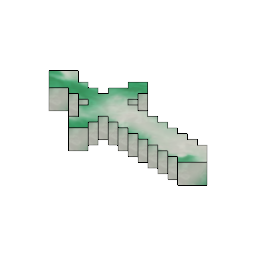
minecraftdiamondsword for big CNC schetch straight_v1 (Autodesk Fusion 360 design; units mm, degrees)
Autodesk Fusion 360 part; units mm, degrees
sketch "big huge diamond sword" plane through (0, 0, 0) normal (0, 0, 1) x (1, 0, 0)
  line L0 (-48.4562, -24.0547) -> (-40.4562, -24.0547)
  line L1 (-40.4562, -24.0547) -> (-40.4562, -16.0547)
  line L2 (-40.4562, -16.0547) -> (-48.4562, -16.0547)
  line L3 (-48.4562, -16.0547) -> (-48.4562, -24.0547)
  line L4 (-40.4562, -24.0547) -> (-32.4562, -24.0547)
  line L5 (-32.4562, -24.0547) -> (-32.4562, -16.0547)
  line L6 (-32.4562, -16.0547) -> (-40.4562, -16.0547)
  line L7 (-40.4562, -16.0547) -> (-40.4562, -24.0547)
  line L8 (-32.4562, -24.0547) -> (-24.4562, -24.0547)
  line L9 (-24.4562, -24.0547) -> (-24.4562, -16.0547)
  line L10 (-32.4562, -16.0547) -> (-32.4562, -24.0547)
  line L11 (-48.4562, -16.0547) -> (-40.4562, -16.0547)
  line L12 (-40.4562, -16.0547) -> (-40.4562, -8.0547)
  line L13 (-40.4562, -8.0547) -> (-48.4562, -8.0547)
  line L14 (-48.4562, -8.0547) -> (-48.4562, -16.0547)
  line L15 (-40.4562, -8.0547) -> (-32.4562, -8.0547)
  line L16 (-32.4562, -8.0547) -> (-32.4562, -16.0547)
  line L17 (-32.4562, -16.0547) -> (-40.4562, -16.0547)
  line L18 (-40.4562, -16.0547) -> (-40.4562, -8.0547)
  line L19 (-48.4562, -8.0547) -> (-40.4562, -8.0547)
  line L20 (-40.4562, -8.0547) -> (-40.4562, -0.0547)
  line L21 (-40.4562, -0.0547) -> (-48.4562, -0.0547)
  line L22 (-48.4562, -0.0547) -> (-48.4562, -8.0547)
  line L23 (-40.4562, -8.0547) -> (-32.4562, -8.0547)
  line L24 (-32.4562, -8.0547) -> (-32.4562, -0.0547)
  line L25 (-32.4562, -0.0547) -> (-40.4562, -0.0547)
  line L26 (-40.4562, -0.0547) -> (-40.4562, -8.0547)
  line L27 (-32.4562, -8.0547) -> (-24.4562, -8.0547)
  line L28 (-24.4562, -8.0547) -> (-24.4562, -16.0547)
  line L29 (-24.4562, -16.0547) -> (-32.4562, -16.0547)
  line L30 (-32.4562, -16.0547) -> (-32.4562, -8.0547)
  line L31 (-32.4562, -8.0547) -> (-24.4562, -8.0547)
  line L32 (-24.4562, -8.0547) -> (-24.4562, -0.0547)
  line L33 (-24.4562, -0.0547) -> (-32.4562, -0.0547)
  line L34 (-32.4562, -0.0547) -> (-32.4562, -8.0547)
  line L35 (-32.4562, -0.0547) -> (-24.4562, -0.0547)
  line L36 (-24.4562, -0.0547) -> (-24.4562, 7.9453)
  line L37 (-24.4562, 7.9453) -> (-32.4562, 7.9453)
  line L38 (-32.4562, 7.9453) -> (-32.4562, -0.0547)
  line L39 (-24.4562, -0.0547) -> (-16.4562, -0.0547)
  line L40 (-16.4562, -0.0547) -> (-16.4562, -8.0547)
  line L41 (-16.4562, -8.0547) -> (-24.4562, -8.0547)
  line L42 (-24.4562, -8.0547) -> (-24.4562, -0.0547)
  line L43 (-24.4562, -0.0547) -> (-16.4562, -0.0547)
  line L44 (-16.4562, -0.0547) -> (-16.4562, 7.9453)
  line L45 (-16.4562, 7.9453) -> (-24.4562, 7.9453)
  line L46 (-24.4562, 7.9453) -> (-24.4562, -0.0547)
  line L47 (-24.4562, 7.9453) -> (-16.4562, 7.9453)
  line L48 (-16.4562, 7.9453) -> (-16.4562, 15.9453)
  line L49 (-16.4562, 15.9453) -> (-24.4562, 15.9453)
  line L50 (-24.4562, 15.9453) -> (-24.4562, 7.9453)
  line L51 (-16.4562, 7.9453) -> (-8.4562, 7.9453)
  line L52 (-8.4562, -0.0547) -> (-16.4562, -0.0547)
  line L53 (-16.4562, -0.0547) -> (-16.4562, 7.9453)
  line L54 (-16.4562, 7.9453) -> (-8.4562, 7.9453)
  line L55 (-8.4562, 7.9453) -> (-8.4562, 15.9453)
  line L56 (-8.4562, 15.9453) -> (-16.4562, 15.9453)
  line L57 (-16.4562, 15.9453) -> (-16.4562, 7.9453)
  line L58 (-16.4562, 15.9453) -> (-8.4562, 15.9453)
  line L59 (-8.4562, 15.9453) -> (-8.4562, 23.9453)
  line L60 (-8.4562, 23.9453) -> (-16.4562, 23.9453)
  line L61 (-16.4562, 23.9453) -> (-16.4562, 15.9453)
  line L62 (-16.4562, 23.9453) -> (-24.4562, 23.9453)
  line L63 (-24.4562, 23.9453) -> (-24.4562, 31.9453)
  line L64 (-24.4562, 31.9453) -> (-16.4562, 31.9453)
  line L65 (-16.4562, 31.9453) -> (-16.4562, 23.9453)
  line L66 (-24.4562, 31.9453) -> (-16.4562, 31.9453)
  line L67 (-16.4562, 31.9453) -> (-16.4562, 39.9453)
  line L68 (-16.4562, 39.9453) -> (-24.4562, 39.9453)
  line L69 (-24.4562, 39.9453) -> (-24.4562, 31.9453)
  line L70 (-24.4562, 39.9453) -> (-32.4562, 39.9453)
  line L71 (-32.4562, 39.9453) -> (-32.4562, 47.9453)
  line L72 (-32.4562, 47.9453) -> (-24.4562, 47.9453)
  line L73 (-24.4562, 47.9453) -> (-24.4562, 39.9453)
  line L74 (-32.4562, 47.9453) -> (-24.4562, 47.9453)
  line L75 (-24.4562, 47.9453) -> (-24.4562, 55.9453)
  line L76 (-24.4562, 55.9453) -> (-32.4562, 55.9453)
  line L77 (-32.4562, 55.9453) -> (-32.4562, 47.9453)
  line L78 (-24.4562, 47.9453) -> (-16.4562, 47.9453)
  line L79 (-16.4562, 47.9453) -> (-16.4562, 55.9453)
  line L80 (-16.4562, 55.9453) -> (-24.4562, 55.9453)
  line L81 (-24.4562, 55.9453) -> (-24.4562, 47.9453)
  line L82 (-24.4562, 39.9453) -> (-16.4562, 39.9453)
  line L83 (-16.4562, 39.9453) -> (-16.4562, 47.9453)
  line L84 (-16.4562, 47.9453) -> (-24.4562, 47.9453)
  line L85 (-24.4562, 47.9453) -> (-24.4562, 39.9453)
  line L86 (-16.4562, 47.9453) -> (-8.4562, 47.9453)
  line L87 (-8.4562, 47.9453) -> (-8.4562, 39.9453)
  line L88 (-8.4562, 39.9453) -> (-16.4562, 39.9453)
  line L89 (-16.4562, 39.9453) -> (-16.4562, 47.9453)
  line L90 (-16.4562, 39.9453) -> (-8.4562, 39.9453)
  line L91 (-8.4562, 39.9453) -> (-8.4562, 31.9453)
  line L92 (-8.4562, 31.9453) -> (-16.4562, 31.9453)
  line L93 (-16.4562, 31.9453) -> (-16.4562, 39.9453)
  line L94 (-16.4562, 23.9453) -> (-8.4562, 23.9453)
  line L95 (-8.4562, 23.9453) -> (-8.4562, 31.9453)
  line L96 (-8.4562, 31.9453) -> (-16.4562, 31.9453)
  line L97 (-16.4562, 31.9453) -> (-16.4562, 23.9453)
  line L98 (-8.4562, 7.9453) -> (-0.4562, 7.9453)
  line L99 (-8.4562, -0.0547) -> (-8.4562, 7.9453)
  line L100 (-8.4562, 15.9453) -> (-0.4562, 15.9453)
  line L101 (-0.4562, 15.9453) -> (-0.4562, 7.9453)
  line L102 (-8.4562, 7.9453) -> (-8.4562, 15.9453)
  line L103 (-8.4562, 23.9453) -> (-0.4562, 23.9453)
  line L104 (-0.4562, 23.9453) -> (-0.4562, 15.9453)
  line L105 (-0.4562, 15.9453) -> (-8.4562, 15.9453)
  line L106 (-8.4562, 15.9453) -> (-8.4562, 23.9453)
  line L107 (-0.4562, 7.9453) -> (7.5438, 7.9453)
  line L108 (7.5438, 7.9453) -> (7.5438, -0.0547)
  line L109 (7.5438, -0.0547) -> (-0.4562, -0.0547)
  line L110 (-0.4562, -0.0547) -> (-0.4562, 7.9453)
  line L111 (-0.4562, 7.9453) -> (7.5438, 7.9453)
  line L112 (7.5438, 7.9453) -> (7.5438, 15.9453)
  line L113 (7.5438, 15.9453) -> (-0.4562, 15.9453)
  line L114 (-0.4562, 15.9453) -> (-0.4562, 7.9453)
  line L115 (7.5438, 7.9453) -> (15.5438, 7.9453)
  line L116 (15.5438, 7.9453) -> (15.5438, -0.0547)
  line L117 (15.5438, -0.0547) -> (7.5438, -0.0547)
  line L118 (7.5438, -0.0547) -> (7.5438, 7.9453)
  line L119 (15.5438, -0.0547) -> (23.5438, -0.0547)
  line L120 (23.5438, -0.0547) -> (23.5438, 7.9453)
  line L121 (23.5438, 7.9453) -> (15.5438, 7.9453)
  line L122 (15.5438, 7.9453) -> (15.5438, -0.0547)
  line L123 (23.5438, -0.0547) -> (31.5438, -0.0547)
  line L124 (31.5438, -0.0547) -> (31.5438, 7.9453)
  line L125 (31.5438, 7.9453) -> (23.5438, 7.9453)
  line L126 (23.5438, 7.9453) -> (23.5438, -0.0547)
  line L127 (15.5438, -0.0547) -> (23.5438, -0.0547)
  line L128 (23.5438, -0.0547) -> (23.5438, -8.0547)
  line L129 (23.5438, -8.0547) -> (15.5438, -8.0547)
  line L130 (15.5438, -8.0547) -> (15.5438, -0.0547)
  line L131 (23.5438, -0.0547) -> (31.5438, -0.0547)
  line L132 (31.5438, -0.0547) -> (31.5438, -8.0547)
  line L133 (31.5438, -8.0547) -> (23.5438, -8.0547)
  line L134 (23.5438, -8.0547) -> (23.5438, -0.0547)
  line L135 (-8.4562, 31.9453) -> (-0.4562, 31.9453)
  line L136 (-0.4562, 31.9453) -> (-0.4562, 23.9453)
  line L137 (-0.4562, 23.9453) -> (-8.4562, 23.9453)
  line L138 (-8.4562, 23.9453) -> (-8.4562, 31.9453)
  line L139 (-0.4562, 23.9453) -> (7.5438, 23.9453)
  line L140 (7.5438, 23.9453) -> (7.5438, 15.9453)
  line L141 (7.5438, 15.9453) -> (-0.4562, 15.9453)
  line L142 (-0.4562, 15.9453) -> (-0.4562, 23.9453)
  line L143 (-8.4562, 39.9453) -> (-0.4562, 39.9453)
  line L144 (-0.4562, 39.9453) -> (-0.4562, 31.9453)
  line L145 (-0.4562, 31.9453) -> (-8.4562, 31.9453)
  line L146 (-8.4562, 31.9453) -> (-8.4562, 39.9453)
  line L147 (-0.4562, 31.9453) -> (7.5438, 31.9453)
  line L148 (7.5438, 31.9453) -> (7.5438, 23.9453)
  line L149 (7.5438, 23.9453) -> (-0.4562, 23.9453)
  line L150 (-0.4562, 23.9453) -> (-0.4562, 31.9453)
  line L151 (-0.4562, 39.9453) -> (7.5438, 39.9453)
  line L152 (7.5438, 39.9453) -> (7.5438, 31.9453)
  line L153 (7.5438, 31.9453) -> (-0.4562, 31.9453)
  line L154 (-0.4562, 31.9453) -> (-0.4562, 39.9453)
  line L155 (7.5438, 15.9453) -> (15.5438, 15.9453)
  line L156 (15.5438, 15.9453) -> (15.5438, 7.9453)
  line L157 (15.5438, 7.9453) -> (7.5438, 7.9453)
  line L158 (7.5438, 7.9453) -> (7.5438, 15.9453)
  line L159 (15.5438, 15.9453) -> (23.5438, 15.9453)
  line L160 (23.5438, 15.9453) -> (23.5438, 7.9453)
  line L161 (23.5438, 7.9453) -> (15.5438, 7.9453)
  line L162 (15.5438, 7.9453) -> (15.5438, 15.9453)
  line L163 (7.5438, 23.9453) -> (15.5438, 23.9453)
  line L164 (15.5438, 23.9453) -> (15.5438, 15.9453)
  line L165 (15.5438, 15.9453) -> (7.5438, 15.9453)
  line L166 (7.5438, 15.9453) -> (7.5438, 23.9453)
  line L167 (7.5438, 31.9453) -> (15.5438, 31.9453)
  line L168 (15.5438, 31.9453) -> (15.5438, 23.9453)
  line L169 (15.5438, 23.9453) -> (7.5438, 23.9453)
  line L170 (7.5438, 23.9453) -> (7.5438, 31.9453)
  line L171 (15.5438, 23.9453) -> (7.5438, 23.9453)
  line L172 (7.5438, 23.9453) -> (7.5438, 31.9453)
  line L173 (7.5438, 31.9453) -> (15.5438, 31.9453)
  line L174 (15.5438, 31.9453) -> (15.5438, 23.9453)
  line L175 (15.5438, 23.9453) -> (23.5438, 23.9453)
  line L176 (23.5438, 23.9453) -> (23.5438, 31.9453)
  line L177 (23.5438, 31.9453) -> (15.5438, 31.9453)
  line L178 (15.5438, 31.9453) -> (15.5438, 23.9453)
  line L179 (7.5438, 31.9453) -> (15.5438, 31.9453)
  line L180 (15.5438, 31.9453) -> (15.5438, 39.9453)
  line L181 (15.5438, 39.9453) -> (7.5438, 39.9453)
  line L182 (7.5438, 39.9453) -> (7.5438, 31.9453)
  line L183 (15.5438, 31.9453) -> (23.5438, 31.9453)
  line L184 (23.5438, 31.9453) -> (23.5438, 39.9453)
  line L185 (23.5438, 39.9453) -> (15.5438, 39.9453)
  line L186 (15.5438, 39.9453) -> (15.5438, 31.9453)
  line L187 (23.5438, 31.9453) -> (31.5438, 31.9453)
  line L188 (31.5438, 31.9453) -> (31.5438, 39.9453)
  line L189 (31.5438, 39.9453) -> (23.5438, 39.9453)
  line L190 (23.5438, 39.9453) -> (23.5438, 31.9453)
  line L191 (-0.4562, 39.9453) -> (7.5438, 39.9453)
  line L192 (7.5438, 39.9453) -> (7.5438, 47.9453)
  line L193 (7.5438, 47.9453) -> (-0.4562, 47.9453)
  line L194 (-0.4562, 47.9453) -> (-0.4562, 39.9453)
  line L195 (7.5438, 39.9453) -> (15.5438, 39.9453)
  line L196 (15.5438, 39.9453) -> (15.5438, 47.9453)
  line L197 (15.5438, 47.9453) -> (7.5438, 47.9453)
  line L198 (7.5438, 47.9453) -> (7.5438, 39.9453)
  line L199 (15.5438, 47.9453) -> (7.5438, 47.9453)
  line L200 (7.5438, 47.9453) -> (7.5438, 55.9453)
  line L201 (7.5438, 55.9453) -> (15.5438, 55.9453)
  line L202 (15.5438, 55.9453) -> (15.5438, 47.9453)
  line L203 (15.5438, 39.9453) -> (23.5438, 39.9453)
  line L204 (23.5438, 39.9453) -> (23.5438, 47.9453)
  line L205 (23.5438, 47.9453) -> (15.5438, 47.9453)
  line L206 (15.5438, 47.9453) -> (15.5438, 39.9453)
  line L207 (15.5438, 47.9453) -> (23.5438, 47.9453)
  line L208 (23.5438, 47.9453) -> (23.5438, 55.9453)
  line L209 (23.5438, 55.9453) -> (15.5438, 55.9453)
  line L210 (15.5438, 55.9453) -> (15.5438, 47.9453)
  line L211 (23.5438, 39.9453) -> (31.5438, 39.9453)
  line L212 (31.5438, 39.9453) -> (31.5438, 47.9453)
  line L213 (31.5438, 47.9453) -> (23.5438, 47.9453)
  line L214 (23.5438, 47.9453) -> (23.5438, 39.9453)
  line L215 (15.5438, 55.9453) -> (23.5438, 55.9453)
  line L216 (23.5438, 55.9453) -> (23.5438, 63.9453)
  line L217 (23.5438, 63.9453) -> (15.5438, 63.9453)
  line L218 (15.5438, 63.9453) -> (15.5438, 55.9453)
  line L219 (31.5438, 39.9453) -> (39.5438, 39.9453)
  line L220 (39.5438, 39.9453) -> (39.5438, 47.9453)
  line L221 (39.5438, 47.9453) -> (31.5438, 47.9453)
  line L222 (31.5438, 47.9453) -> (31.5438, 39.9453)
  line L223 (23.5438, 47.9453) -> (31.5438, 47.9453)
  line L224 (31.5438, 47.9453) -> (31.5438, 55.9453)
  line L225 (31.5438, 55.9453) -> (23.5438, 55.9453)
  line L226 (23.5438, 55.9453) -> (23.5438, 47.9453)
  line L227 (31.5438, 55.9453) -> (39.5438, 55.9453)
  line L228 (39.5438, 55.9453) -> (39.5438, 63.9453)
  line L229 (39.5438, 63.9453) -> (31.5438, 63.9453)
  line L230 (31.5438, 63.9453) -> (31.5438, 55.9453)
  line L231 (31.5438, 55.9453) -> (23.5438, 55.9453)
  line L232 (23.5438, 55.9453) -> (23.5438, 63.9453)
  line L233 (23.5438, 63.9453) -> (31.5438, 63.9453)
  line L234 (31.5438, 63.9453) -> (31.5438, 55.9453)
  line L235 (31.5438, 55.9453) -> (39.5438, 55.9453)
  line L236 (39.5438, 55.9453) -> (39.5438, 47.9453)
  line L237 (39.5438, 47.9453) -> (31.5438, 47.9453)
  line L238 (31.5438, 47.9453) -> (31.5438, 55.9453)
  line L239 (23.5438, 63.9453) -> (31.5438, 63.9453)
  line L240 (31.5438, 63.9453) -> (31.5438, 71.9453)
  line L241 (31.5438, 71.9453) -> (23.5438, 71.9453)
  line L242 (23.5438, 71.9453) -> (23.5438, 63.9453)
  line L243 (31.5438, 63.9453) -> (39.5438, 63.9453)
  line L244 (39.5438, 63.9453) -> (39.5438, 71.9453)
  line L245 (39.5438, 71.9453) -> (31.5438, 71.9453)
  line L246 (31.5438, 71.9453) -> (31.5438, 63.9453)
  line L247 (39.5438, 47.9453) -> (47.5438, 47.9453)
  line L248 (47.5438, 47.9453) -> (47.5438, 55.9453)
  line L249 (47.5438, 55.9453) -> (39.5438, 55.9453)
  line L250 (39.5438, 55.9453) -> (39.5438, 47.9453)
  line L251 (39.5438, 55.9453) -> (47.5438, 55.9453)
  line L252 (47.5438, 55.9453) -> (47.5438, 63.9453)
  line L253 (47.5438, 63.9453) -> (39.5438, 63.9453)
  line L254 (39.5438, 63.9453) -> (39.5438, 55.9453)
  line L255 (39.5438, 63.9453) -> (47.5438, 63.9453)
  line L256 (47.5438, 63.9453) -> (47.5438, 71.9453)
  line L257 (47.5438, 71.9453) -> (39.5438, 71.9453)
  line L258 (39.5438, 71.9453) -> (39.5438, 63.9453)
  line L259 (31.5438, 71.9453) -> (39.5438, 71.9453)
  line L260 (39.5438, 71.9453) -> (39.5438, 79.9453)
  line L261 (39.5438, 79.9453) -> (31.5438, 79.9453)
  line L262 (31.5438, 79.9453) -> (31.5438, 71.9453)
  line L263 (47.5438, 55.9453) -> (55.5438, 55.9453)
  line L264 (55.5438, 55.9453) -> (55.5438, 63.9453)
  line L265 (55.5438, 63.9453) -> (47.5438, 63.9453)
  line L266 (47.5438, 63.9453) -> (47.5438, 55.9453)
  line L267 (39.5438, 71.9453) -> (47.5438, 71.9453)
  line L268 (47.5438, 71.9453) -> (47.5438, 79.9453)
  line L269 (47.5438, 79.9453) -> (39.5438, 79.9453)
  line L270 (39.5438, 79.9453) -> (39.5438, 71.9453)
  line L271 (47.5438, 63.9453) -> (55.5438, 63.9453)
  line L272 (55.5438, 63.9453) -> (55.5438, 71.9453)
  line L273 (55.5438, 71.9453) -> (47.5438, 71.9453)
  line L274 (47.5438, 71.9453) -> (47.5438, 63.9453)
  line L275 (47.5438, 71.9453) -> (55.5438, 71.9453)
  line L276 (55.5438, 71.9453) -> (55.5438, 79.9453)
  line L277 (55.5438, 79.9453) -> (47.5438, 79.9453)
  line L278 (47.5438, 79.9453) -> (47.5438, 71.9453)
  line L279 (55.5438, 63.9453) -> (63.5438, 63.9453)
  line L280 (63.5438, 63.9453) -> (63.5438, 71.9453)
  line L281 (63.5438, 71.9453) -> (55.5438, 71.9453)
  line L282 (55.5438, 71.9453) -> (55.5438, 63.9453)
  line L283 (39.5438, 79.9453) -> (47.5438, 79.9453)
  line L284 (47.5438, 79.9453) -> (47.5438, 87.9453)
  line L285 (47.5438, 87.9453) -> (39.5438, 87.9453)
  line L286 (39.5438, 87.9453) -> (39.5438, 79.9453)
  line L287 (55.5438, 79.9453) -> (63.5438, 79.9453)
  line L288 (63.5438, 79.9453) -> (63.5438, 71.9453)
  line L289 (63.5438, 71.9453) -> (55.5438, 71.9453)
  line L290 (55.5438, 71.9453) -> (55.5438, 79.9453)
  line L291 (47.5438, 79.9453) -> (55.5438, 79.9453)
  line L292 (55.5438, 79.9453) -> (55.5438, 87.9453)
  line L293 (55.5438, 87.9453) -> (47.5438, 87.9453)
  line L294 (47.5438, 87.9453) -> (47.5438, 79.9453)
  line L295 (55.5438, 79.9453) -> (63.5438, 79.9453)
  line L296 (63.5438, 79.9453) -> (63.5438, 87.9453)
  line L297 (63.5438, 87.9453) -> (55.5438, 87.9453)
  line L298 (55.5438, 87.9453) -> (55.5438, 79.9453)
  line L299 (63.5438, 71.9453) -> (71.5438, 71.9453)
  line L300 (71.5438, 71.9453) -> (71.5438, 79.9453)
  line L301 (71.5438, 79.9453) -> (63.5438, 79.9453)
  line L302 (63.5438, 79.9453) -> (63.5438, 71.9453)
  line L303 (47.5438, 87.9453) -> (55.5438, 87.9453)
  line L304 (55.5438, 87.9453) -> (55.5438, 95.9453)
  line L305 (55.5438, 95.9453) -> (47.5438, 95.9453)
  line L306 (47.5438, 95.9453) -> (47.5438, 87.9453)
  line L307 (55.5438, 95.9453) -> (63.5438, 95.9453)
  line L308 (63.5438, 95.9453) -> (63.5438, 87.9453)
  line L309 (63.5438, 87.9453) -> (55.5438, 87.9453)
  line L310 (55.5438, 87.9453) -> (55.5438, 95.9453)
  line L311 (63.5438, 79.9453) -> (71.5438, 79.9453)
  line L312 (71.5438, 79.9453) -> (71.5438, 87.9453)
  line L313 (71.5438, 87.9453) -> (63.5438, 87.9453)
  line L314 (63.5438, 87.9453) -> (63.5438, 79.9453)
  line L315 (63.5438, 87.9453) -> (71.5438, 87.9453)
  line L316 (71.5438, 87.9453) -> (71.5438, 95.9453)
  line L317 (71.5438, 95.9453) -> (63.5438, 95.9453)
  line L318 (63.5438, 95.9453) -> (63.5438, 87.9453)
  line L319 (55.5438, 95.9453) -> (63.5438, 95.9453)
  line L320 (63.5438, 95.9453) -> (63.5438, 103.9453)
  line L321 (63.5438, 103.9453) -> (55.5438, 103.9453)
  line L322 (55.5438, 103.9453) -> (55.5438, 95.9453)
  line L323 (63.5438, 95.9453) -> (71.5438, 95.9453)
  line L324 (71.5438, 95.9453) -> (71.5438, 103.9453)
  line L325 (71.5438, 103.9453) -> (63.5438, 103.9453)
  line L326 (63.5438, 103.9453) -> (63.5438, 95.9453)
  line L327 (71.5438, 79.9453) -> (79.5438, 79.9453)
  line L328 (79.5438, 79.9453) -> (79.5438, 87.9453)
  line L329 (79.5438, 87.9453) -> (71.5438, 87.9453)
  line L330 (71.5438, 87.9453) -> (71.5438, 79.9453)
  line L331 (71.5438, 87.9453) -> (79.5438, 87.9453)
  line L332 (79.5438, 87.9453) -> (79.5438, 95.9453)
  line L333 (79.5438, 95.9453) -> (71.5438, 95.9453)
  line L334 (71.5438, 95.9453) -> (71.5438, 87.9453)
  line L335 (71.5438, 95.9453) -> (63.5438, 95.9453)
  line L336 (63.5438, 95.9453) -> (63.5438, 103.9453)
  line L337 (63.5438, 103.9453) -> (71.5438, 103.9453)
  line L338 (71.5438, 103.9453) -> (71.5438, 95.9453)
  line L339 (71.5438, 95.9453) -> (79.5438, 95.9453)
  line L340 (79.5438, 95.9453) -> (79.5438, 103.9453)
  line L341 (79.5438, 103.9453) -> (71.5438, 103.9453)
  line L342 (71.5438, 103.9453) -> (71.5438, 95.9453)
  dimension "d249" = 8
  dimension "d250" = 8
  dimension "d251" = 8
  dimension "d252" = 8
  dimension "d253" = 8
  dimension "d254" = 8
  dimension "d255" = 8
  dimension "d256" = 8
  dimension "d261" = 8
  dimension "d262" = 8
  dimension "d263" = 8
  dimension "d264" = 8
  dimension "d265" = 8
  dimension "d266" = 8
  dimension "d267" = 8
  dimension "d268" = 8
  dimension "d271" = 8
  dimension "d272" = 8
  dimension "d273" = 8
  dimension "d274" = 8
  dimension "d275" = 8
  dimension "d276" = 8
  dimension "d277" = 8
  dimension "d278" = 8
  dimension "d279" = 8
  dimension "d280" = 8
  dimension "d281" = 8
  dimension "d282" = 8
  dimension "d283" = 8
  dimension "d284" = 8
  dimension "d285" = 8
  dimension "d286" = 8
  dimension "d287" = 8
  dimension "d288" = 8
  dimension "d289" = 8
  dimension "d290" = 8
  dimension "d291" = 8
  dimension "d292" = 8
  dimension "d293" = 8
  dimension "d294" = 8
  dimension "d295" = 8
  dimension "d296" = 8
  dimension "d297" = 8
  dimension "d298" = 8
  dimension "d299" = 8
  dimension "d300" = 8
  dimension "d301" = 8
  dimension "d302" = 8
  dimension "d303" = 8
  dimension "d304" = 8
  dimension "d309" = 8
  dimension "d310" = 8
  dimension "d311" = 8
  dimension "d312" = 8
  dimension "d313" = 8
  dimension "d314" = 8
  dimension "d315" = 8
  dimension "d316" = 8
  dimension "d319" = 8
  dimension "d320" = 8
  dimension "d321" = 8
  dimension "d322" = 8
  dimension "d323" = 8
  dimension "d324" = 8
  dimension "d325" = 8
  dimension "d326" = 8
  dimension "d327" = 8
  dimension "d328" = 8
  dimension "d329" = 8
  dimension "d330" = 8
  dimension "d331" = 8
  dimension "d332" = 8
  dimension "d333" = 8
  dimension "d334" = 8
  dimension "d335" = 8
  dimension "d336" = 8
  dimension "d337" = 8
  dimension "d338" = 8
  dimension "d339" = 8
  dimension "d340" = 8
  dimension "d341" = 8
  dimension "d342" = 8
  dimension "d343" = 8
  dimension "d344" = 8
  dimension "d345" = 8
  dimension "d346" = 8
  dimension "d347" = 8
  dimension "d348" = 8
  dimension "d349" = 8
  dimension "d350" = 8
  dimension "d351" = 8
  dimension "d352" = 8
  dimension "d353" = 8
  dimension "d354" = 8
  dimension "d355" = 8
  dimension "d356" = 8
  dimension "d357" = 8
  dimension "d358" = 8
  dimension "d359" = 8
  dimension "d360" = 8
  dimension "d361" = 8
  dimension "d362" = 8
  dimension "d363" = 8
  dimension "d364" = 8
  dimension "d365" = 8
  dimension "d366" = 8
  dimension "d367" = 8
  dimension "d368" = 8
  dimension "d369" = 8
  dimension "d370" = 8
  dimension "d371" = 8
  dimension "d372" = 8
  dimension "d373" = 8
  dimension "d374" = 8
  dimension "d375" = 8
  dimension "d376" = 8
  dimension "d377" = 8
  dimension "d378" = 8
  dimension "d379" = 8
  dimension "d380" = 8
  dimension "d381" = 8
  dimension "d382" = 8
  dimension "d383" = 8
  dimension "d384" = 8
  dimension "d385" = 8
  dimension "d386" = 8
  dimension "d387" = 8
  dimension "d388" = 8
  dimension "d389" = 8
  dimension "d390" = 8
  dimension "d391" = 8
  dimension "d392" = 8
  dimension "d393" = 8
  dimension "d394" = 8
  dimension "d395" = 8
  dimension "d396" = 8
  dimension "d397" = 8
  dimension "d398" = 8
  dimension "d399" = 8
  dimension "d400" = 8
  dimension "d401" = 8
  dimension "d402" = 8
  dimension "d403" = 8
  dimension "d404" = 8
  dimension "d405" = 8
  dimension "d406" = 8
  dimension "d407" = 8
  dimension "d408" = 8
  dimension "d409" = 8
  dimension "d410" = 8
  dimension "d411" = 8
  dimension "d412" = 8
  dimension "d413" = 8
  dimension "d414" = 8
  dimension "d415" = 8
  dimension "d416" = 8
  dimension "d417" = 8
  dimension "d418" = 8
  dimension "d419" = 8
  dimension "d420" = 8
  dimension "d421" = 8
  dimension "d422" = 8
  dimension "d423" = 8
  dimension "d424" = 8
  dimension "d425" = 8
  dimension "d426" = 8
  dimension "d427" = 8
  dimension "d428" = 8
  dimension "d429" = 8
  dimension "d430" = 8
  dimension "d431" = 8
  dimension "d432" = 8
  dimension "d433" = 8
  dimension "d434" = 8
  constraint horizontal L0
  constraint vertical L1
  constraint horizontal L2
  constraint vertical L3
  constraint horizontal L4
  constraint vertical L5
  constraint horizontal L6
  constraint vertical L7
  constraint horizontal L8
  constraint vertical L9
  constraint vertical L10
  constraint horizontal L11
  constraint vertical L12
  constraint horizontal L13
  constraint vertical L14
  constraint horizontal L15
  constraint vertical L16
  constraint horizontal L17
  constraint vertical L18
  constraint horizontal L19
  constraint vertical L20
  constraint horizontal L21
  constraint vertical L22
  constraint horizontal L23
  constraint vertical L24
  constraint horizontal L25
  constraint vertical L26
  constraint horizontal L27
  constraint vertical L28
  constraint horizontal L29
  constraint vertical L30
  constraint horizontal L31
  constraint vertical L32
  constraint horizontal L33
  constraint vertical L34
  constraint horizontal L35
  constraint vertical L36
  constraint horizontal L37
  constraint vertical L38
  constraint horizontal L39
  constraint vertical L40
  constraint horizontal L41
  constraint vertical L42
  constraint horizontal L43
  constraint vertical L44
  constraint horizontal L45
  constraint vertical L46
  constraint horizontal L47
  constraint vertical L48
  constraint horizontal L49
  constraint vertical L50
  constraint horizontal L51
  constraint horizontal L52
  constraint vertical L53
  constraint horizontal L54
  constraint vertical L55
  constraint horizontal L56
  constraint vertical L57
  constraint horizontal L58
  constraint vertical L59
  constraint horizontal L60
  constraint vertical L61
  constraint horizontal L62
  constraint vertical L63
  constraint horizontal L64
  constraint vertical L65
  constraint horizontal L66
  constraint vertical L67
  constraint horizontal L68
  constraint vertical L69
  constraint horizontal L70
  constraint vertical L71
  constraint horizontal L72
  constraint vertical L73
  constraint vertical L75
  constraint perpendicular L74 L75
  constraint horizontal L76
  constraint parallel L75 L77
  constraint vertical L79
  constraint perpendicular L78 L79
  constraint horizontal L80
  constraint parallel L79 L81
  constraint horizontal L82
  constraint vertical L83
  constraint horizontal L84
  constraint vertical L85
  constraint vertical L87
  constraint perpendicular L86 L87
  constraint horizontal L88
  constraint parallel L87 L89
  constraint horizontal L90
  constraint vertical L91
  constraint horizontal L92
  constraint vertical L93
  constraint horizontal L94
  constraint vertical L95
  constraint horizontal L96
  constraint vertical L97
  constraint horizontal L100
  constraint vertical L101
  constraint vertical L102
  constraint vertical L104
  constraint perpendicular L103 L104
  constraint horizontal L105
  constraint parallel L104 L106
  constraint horizontal L107
  constraint vertical L108
  constraint horizontal L109
  constraint vertical L110
  constraint perpendicular L52 L99
  constraint horizontal L98
  constraint coincident L98.end L101.end
  constraint horizontal L111
  constraint vertical L112
  constraint horizontal L113
  constraint vertical L114
  constraint vertical L116
  constraint perpendicular L115 L116
  constraint horizontal L117
  constraint parallel L116 L118
  constraint horizontal L119
  constraint vertical L120
  constraint horizontal L121
  constraint vertical L122
  constraint vertical L124
  constraint perpendicular L123 L124
  constraint horizontal L125
  constraint parallel L124 L126
  constraint vertical L128
  constraint perpendicular L127 L128
  constraint horizontal L129
  constraint parallel L128 L130
  constraint vertical L132
  constraint perpendicular L131 L132
  constraint horizontal L133
  constraint parallel L132 L134
  constraint vertical L136
  constraint perpendicular L135 L136
  constraint horizontal L137
  constraint parallel L136 L138
  constraint vertical L140
  constraint perpendicular L139 L140
  constraint horizontal L141
  constraint parallel L140 L142
  constraint vertical L144
  constraint perpendicular L143 L144
  constraint horizontal L145
  constraint parallel L144 L146
  constraint vertical L148
  constraint perpendicular L147 L148
  constraint horizontal L149
  constraint parallel L148 L150
  constraint vertical L152
  constraint perpendicular L151 L152
  constraint horizontal L153
  constraint parallel L152 L154
  constraint vertical L156
  constraint perpendicular L155 L156
  constraint horizontal L157
  constraint parallel L156 L158
  constraint vertical L160
  constraint perpendicular L159 L160
  constraint horizontal L161
  constraint parallel L160 L162
  constraint vertical L164
  constraint perpendicular L163 L164
  constraint horizontal L165
  constraint parallel L164 L166
  constraint vertical L168
  constraint perpendicular L167 L168
  constraint horizontal L169
  constraint parallel L168 L170
  constraint vertical L172
  constraint perpendicular L171 L172
  constraint horizontal L173
  constraint parallel L172 L174
  constraint vertical L176
  constraint perpendicular L175 L176
  constraint horizontal L177
  constraint parallel L176 L178
  constraint vertical L180
  constraint perpendicular L179 L180
  constraint horizontal L181
  constraint parallel L180 L182
  constraint vertical L184
  constraint perpendicular L183 L184
  constraint horizontal L185
  constraint parallel L184 L186
  constraint vertical L188
  constraint perpendicular L187 L188
  constraint horizontal L189
  constraint parallel L188 L190
  constraint horizontal L191
  constraint vertical L192
  constraint horizontal L193
  constraint vertical L194
  constraint vertical L196
  constraint perpendicular L195 L196
  constraint horizontal L197
  constraint parallel L196 L198
  constraint vertical L200
  constraint perpendicular L199 L200
  constraint horizontal L201
  constraint parallel L200 L202
  constraint vertical L204
  constraint perpendicular L203 L204
  constraint horizontal L205
  constraint parallel L204 L206
  constraint horizontal L207
  constraint vertical L208
  constraint horizontal L209
  constraint vertical L210
  constraint vertical L212
  constraint perpendicular L211 L212
  constraint horizontal L213
  constraint parallel L212 L214
  constraint vertical L216
  constraint perpendicular L215 L216
  constraint horizontal L217
  constraint parallel L216 L218
  constraint vertical L220
  constraint perpendicular L219 L220
  constraint horizontal L221
  constraint parallel L220 L222
  constraint vertical L224
  constraint perpendicular L223 L224
  constraint horizontal L225
  constraint parallel L224 L226
  constraint vertical L228
  constraint perpendicular L227 L228
  constraint horizontal L229
  constraint parallel L228 L230
  constraint vertical L232
  constraint perpendicular L231 L232
  constraint horizontal L233
  constraint parallel L232 L234
  constraint vertical L236
  constraint perpendicular L235 L236
  constraint horizontal L237
  constraint parallel L236 L238
  constraint vertical L240
  constraint perpendicular L239 L240
  constraint horizontal L241
  constraint parallel L240 L242
  constraint vertical L244
  constraint perpendicular L243 L244
  constraint horizontal L245
  constraint parallel L244 L246
  constraint vertical L248
  constraint perpendicular L247 L248
  constraint horizontal L249
  constraint parallel L248 L250
  constraint vertical L252
  constraint perpendicular L251 L252
  constraint horizontal L253
  constraint parallel L252 L254
  constraint vertical L256
  constraint perpendicular L255 L256
  constraint horizontal L257
  constraint parallel L256 L258
  constraint vertical L260
  constraint perpendicular L259 L260
  constraint horizontal L261
  constraint parallel L260 L262
  constraint vertical L264
  constraint perpendicular L263 L264
  constraint horizontal L265
  constraint parallel L264 L266
  constraint vertical L268
  constraint perpendicular L267 L268
  constraint horizontal L269
  constraint parallel L268 L270
  constraint horizontal L271
  constraint vertical L272
  constraint horizontal L273
  constraint vertical L274
  constraint vertical L276
  constraint perpendicular L275 L276
  constraint horizontal L277
  constraint parallel L276 L278
  constraint vertical L280
  constraint perpendicular L279 L280
  constraint horizontal L281
  constraint parallel L280 L282
  constraint vertical L284
  constraint perpendicular L283 L284
  constraint horizontal L285
  constraint parallel L284 L286
  constraint vertical L288
  constraint perpendicular L287 L288
  constraint horizontal L289
  constraint parallel L288 L290
  constraint vertical L292
  constraint perpendicular L291 L292
  constraint horizontal L293
  constraint parallel L292 L294
  constraint horizontal L295
  constraint vertical L296
  constraint horizontal L297
  constraint vertical L298
  constraint horizontal L299
  constraint vertical L300
  constraint horizontal L301
  constraint vertical L302
  constraint vertical L304
  constraint perpendicular L303 L304
  constraint horizontal L305
  constraint parallel L304 L306
  constraint horizontal L307
  constraint vertical L308
  constraint horizontal L309
  constraint vertical L310
  constraint horizontal L311
  constraint vertical L312
  constraint horizontal L313
  constraint vertical L314
  constraint horizontal L315
  constraint vertical L316
  constraint horizontal L317
  constraint vertical L318
  constraint horizontal L319
  constraint vertical L320
  constraint horizontal L321
  constraint vertical L322
  constraint horizontal L323
  constraint vertical L324
  constraint horizontal L325
  constraint vertical L326
  constraint horizontal L327
  constraint vertical L328
  constraint horizontal L329
  constraint vertical L330
  constraint horizontal L331
  constraint vertical L332
  constraint horizontal L333
  constraint vertical L334
  constraint horizontal L335
  constraint vertical L336
  constraint horizontal L337
  constraint vertical L338
  constraint vertical L340
  constraint perpendicular L339 L340
  constraint horizontal L341
  constraint parallel L340 L342
  measures "d249" distance of L0.start L0.end
  measures "d250" distance of L0.start L2.end
  measures "d251" distance of L0.end L4.end
  measures "d252" distance of L0.end L1.end
  measures "d253" distance of L4.end L8.end
  measures "d254" distance of L4.end L5.end
  measures "d255" distance of L2.end L1.end
  measures "d256" distance of L2.end L13.end
  measures "d261" distance of L12.end L15.end
  measures "d262" distance of L12.end L1.end
  measures "d263" distance of L13.end L12.end
  measures "d264" distance of L13.end L21.end
  measures "d265" distance of L12.end L15.end
  measures "d266" distance of L12.end L20.end
  measures "d267" distance of L15.end L27.end
  measures "d268" distance of L15.end L5.end
  measures "d271" distance of L15.end L27.end
  measures "d272" distance of L15.end L24.end
  measures "d273" distance of L24.end L32.end
  measures "d274" distance of L24.end L37.end
  measures "d275" distance of L32.end L39.end
  measures "d276" distance of L32.end L27.end
  measures "d277" distance of L32.end L39.end
  measures "d278" distance of L32.end L36.end
  measures "d279" distance of L36.end L44.end
  measures "d280" distance of L36.end L49.end
  measures "d281" distance of L44.end L51.end
  measures "d282" distance of L44.end L39.end
  measures "d283" distance of L44.end L51.end
  measures "d284" distance of L44.end L48.end
  measures "d285" distance of L48.end L55.end
  measures "d286" distance of L48.end L60.end
  measures "d287" distance of L60.end L62.end
  measures "d288" distance of L60.end L64.end
  measures "d289" distance of L63.end L64.end
  measures "d290" distance of L63.end L68.end
  measures "d291" distance of L68.end L70.end
  measures "d292" distance of L68.end L72.end
  measures "d293" distance of L71.end L72.end
  measures "d294" distance of L71.end L76.end
  measures "d295" distance of L72.end L78.end
  measures "d296" distance of L72.end L75.end
  measures "d297" distance of L68.end L67.end
  measures "d298" distance of L68.end L72.end
  measures "d299" distance of L78.end L86.end
  measures "d300" distance of L78.end L67.end
  measures "d301" distance of L67.end L87.end
  measures "d302" distance of L67.end L64.end
  measures "d303" distance of L60.end L59.end
  measures "d304" distance of L60.end L64.end
  measures "d309" distance of L51.end L98.end
  measures "d310" distance of L51.end L52.start
  measures "d311" distance of L55.end L100.end
  measures "d312" distance of L55.end L51.end
  measures "d313" distance of L59.end L103.end
  measures "d314" distance of L59.end L55.end
  measures "d315" distance of L98.end L107.end
  measures "d316" distance of L98.end L109.end
  measures "d319" distance of L98.end L107.end
  measures "d320" distance of L98.end L100.end
  measures "d321" distance of L107.end L115.end
  measures "d322" distance of L107.end L108.end
  measures "d323" distance of L116.end L119.end
  measures "d324" distance of L116.end L115.end
  measures "d325" distance of L119.end L123.end
  measures "d326" distance of L119.end L120.end
  measures "d327" distance of L116.end L119.end
  measures "d328" distance of L116.end L129.end
  measures "d329" distance of L119.end L123.end
  measures "d330" distance of L119.end L128.end
  measures "d331" distance of L91.end L135.end
  measures "d332" distance of L91.end L59.end
  measures "d333" distance of L103.end L139.end
  measures "d334" distance of L103.end L100.end
  measures "d335" distance of L87.end L143.end
  measures "d336" distance of L87.end L91.end
  measures "d337" distance of L135.end L147.end
  measures "d338" distance of L135.end L103.end
  measures "d339" distance of L143.end L151.end
  measures "d340" distance of L143.end L135.end
  measures "d341" distance of L112.end L155.end
  measures "d342" distance of L112.end L107.end
  measures "d343" distance of L155.end L159.end
  measures "d344" distance of L155.end L115.end
  measures "d345" distance of L139.end L163.end
  measures "d346" distance of L139.end L112.end
  measures "d347" distance of L147.end L167.end
  measures "d348" distance of L147.end L139.end
  measures "d349" distance of L163.end L139.end
  measures "d350" distance of L163.end L167.end
  measures "d351" distance of L163.end L175.end
  measures "d352" distance of L163.end L167.end
  measures "d353" distance of L147.end L167.end
  measures "d354" distance of L147.end L151.end
  measures "d355" distance of L167.end L176.end
  measures "d356" distance of L167.end L180.end
  measures "d357" distance of L176.end L187.end
  measures "d358" distance of L176.end L184.end
  measures "d359" distance of L143.end L151.end
  measures "d360" distance of L143.end L193.end
  measures "d361" distance of L151.end L180.end
  measures "d362" distance of L151.end L192.end
  measures "d363" distance of L196.end L192.end
  measures "d364" distance of L196.end L201.end
  measures "d365" distance of L180.end L184.end
  measures "d366" distance of L180.end L196.end
  measures "d367" distance of L196.end L204.end
  measures "d368" distance of L196.end L201.end
  measures "d369" distance of L184.end L188.end
  measures "d370" distance of L184.end L204.end
  measures "d371" distance of L201.end L208.end
  measures "d372" distance of L201.end L217.end
  measures "d373" distance of L188.end L219.end
  measures "d374" distance of L188.end L212.end
  measures "d375" distance of L204.end L212.end
  measures "d376" distance of L204.end L208.end
  measures "d377" distance of L224.end L227.end
  measures "d378" distance of L224.end L229.end
  measures "d379" distance of L224.end L208.end
  measures "d380" distance of L224.end L229.end
  measures "d381" distance of L224.end L227.end
  measures "d382" distance of L224.end L212.end
  measures "d383" distance of L216.end L229.end
  measures "d384" distance of L216.end L241.end
  measures "d385" distance of L229.end L228.end
  measures "d386" distance of L229.end L240.end
  measures "d387" distance of L220.end L247.end
  measures "d388" distance of L220.end L227.end
  measures "d389" distance of L227.end L248.end
  measures "d390" distance of L227.end L228.end
  measures "d391" distance of L228.end L252.end
  measures "d392" distance of L228.end L244.end
  measures "d393" distance of L240.end L244.end
  measures "d394" distance of L240.end L261.end
  measures "d395" distance of L248.end L263.end
  measures "d396" distance of L248.end L252.end
  measures "d397" distance of L244.end L256.end
  measures "d398" distance of L244.end L260.end
  measures "d399" distance of L252.end L264.end
  measures "d400" distance of L252.end L256.end
  measures "d401" distance of L256.end L272.end
  measures "d402" distance of L256.end L268.end
  measures "d403" distance of L264.end L279.end
  measures "d404" distance of L264.end L272.end
  measures "d405" distance of L260.end L268.end
  measures "d406" distance of L260.end L285.end
  measures "d407" distance of L276.end L287.end
  measures "d408" distance of L276.end L272.end
  measures "d409" distance of L268.end L276.end
  measures "d410" distance of L268.end L284.end
  measures "d411" distance of L276.end L287.end
  measures "d412" distance of L276.end L292.end
  measures "d413" distance of L280.end L299.end
  measures "d414" distance of L280.end L287.end
  measures "d415" distance of L284.end L292.end
  measures "d416" distance of L284.end L305.end
  measures "d417" distance of L304.end L307.end
  measures "d418" distance of L304.end L292.end
  measures "d419" distance of L287.end L300.end
  measures "d420" distance of L287.end L296.end
  measures "d421" distance of L296.end L312.end
  measures "d422" distance of L296.end L307.end
  measures "d423" distance of L304.end L307.end
  measures "d424" distance of L304.end L321.end
  measures "d425" distance of L307.end L316.end
  measures "d426" distance of L307.end L320.end
  measures "d427" distance of L300.end L327.end
  measures "d428" distance of L300.end L312.end
  measures "d429" distance of L312.end L328.end
  measures "d430" distance of L312.end L316.end
  measures "d431" distance of L316.end L307.end
  measures "d432" distance of L316.end L324.end
  measures "d433" distance of L316.end L332.end
  measures "d434" distance of L316.end L324.end
extrude "Extrude11" add sketch "big huge diamond sword" along normal blind 23 makes body 1
sketch "board prepare" plane through (0, 0, 0) normal (0, 0, 1) x (1, 0, 0)
  line L0 (0, 0) -> (310, 0)
  line L1 (310, 0) -> (310, 124)
  line L2 (310, 124) -> (0, 124)
  line L3 (0, 124) -> (0, 0)
  dimension "d437" = 310
  dimension "d438" = 124
  constraint horizontal L0
  constraint vertical L1
  constraint horizontal L2
  constraint vertical L3
  constraint coincident L0.start L3.end
  measures "d437" distance of L0.start L0.end
  measures "d438" distance of L0.start L2.end
extrude "Extrude12" add sketch "board prepare" along normal blind 23 separate body makes body 2
move_body "Move2" bodies 1 to x (0.707107, -0.707107, 0) y (0.707107, 0.707107, 0) z (0, 0, 1) at (0, 0, 0)
move_body "Move3" bodies 1 to x (1, 0, 0) y (0, 1, 0) z (0, 0, 1) at (136.2, 74.374, -13.1911)
move_body "Move4" bodies 1 to x (1, 0, 0) y (0, 1, 0) z (0, 0, 1) at (-18.4783, -46.3736, -19.9999)
move_body "Move5" bodies 1 to x (1, 0, 0) y (0, 1, 0) z (0, 0, 1) at (-66.4487, 7.3542, 0)
move_body "Move6" bodies 1 to x (1, 0, 0) y (0, 1, 0) z (0, 0, 1) at (0, 0, 33.191)
move_body "Move7" bodies 1 to x (1, 0, 0) y (0, 1, 0) z (0, 0, 1) at (-0.0003, -7.3542, 0)
equation "d = 8 mm"
equation "StockHeight = 23 mm"
equation "d249 = d"
equation "d250 = d"
equation "d251 = d"
equation "d252 = d"
equation "d253 = d"
equation "d254 = d"
equation "d255 = d"
equation "d256 = d"
equation "d261 = d"
equation "d262 = d"
equation "d263 = d"
equation "d264 = d"
equation "d265 = d"
equation "d266 = d"
equation "d267 = d"
equation "d268 = d"
equation "d271 = d"
equation "d272 = d"
equation "d273 = d"
equation "d274 = d"
equation "d275 = d"
equation "d276 = d"
equation "d277 = d"
equation "d278 = d"
equation "d279 = d"
equation "d280 = d"
equation "d281 = d"
equation "d282 = d"
equation "d283 = d"
equation "d284 = d"
equation "d285 = d"
equation "d286 = d"
equation "d287 = d"
equation "d288 = d"
equation "d289 = d"
equation "d290 = d"
equation "d291 = d"
equation "d292 = d"
equation "d293 = d"
equation "d294 = d"
equation "d295 = d"
equation "d296 = d"
equation "d297 = d"
equation "d298 = d"
equation "d299 = d"
equation "d300 = d"
equation "d301 = d"
equation "d302 = d"
equation "d303 = d"
equation "d304 = d"
equation "d309 = d"
equation "d310 = d"
equation "d311 = d"
equation "d312 = d"
equation "d313 = d"
equation "d314 = d"
equation "d315 = d"
equation "d316 = d"
equation "d319 = d"
equation "d320 = d"
equation "d321 = d"
equation "d322 = d"
equation "d323 = d"
equation "d324 = d"
equation "d325 = d"
equation "d326 = d"
equation "d327 = d"
equation "d328 = d"
equation "d329 = d"
equation "d330 = d"
equation "d331 = d"
equation "d332 = d"
equation "d333 = d"
equation "d334 = d"
equation "d335 = d"
equation "d336 = d"
equation "d337 = d"
equation "d338 = d"
equation "d339 = d"
equation "d340 = d"
equation "d341 = d"
equation "d342 = d"
equation "d343 = d"
equation "d344 = d"
equation "d345 = d"
equation "d346 = d"
equation "d347 = d"
equation "d348 = d"
equation "d349 = d"
equation "d350 = d"
equation "d351 = d"
equation "d352 = d"
equation "d353 = d"
equation "d354 = d"
equation "d355 = d"
equation "d356 = d"
equation "d357 = d"
equation "d358 = d"
equation "d359 = d"
equation "d360 = d"
equation "d361 = d"
equation "d362 = d"
equation "d363 = d"
equation "d364 = d"
equation "d365 = d"
equation "d366 = d"
equation "d367 = d"
equation "d368 = d"
equation "d369 = d"
equation "d370 = d"
equation "d371 = d"
equation "d372 = d"
equation "d373 = d"
equation "d374 = d"
equation "d375 = d"
equation "d376 = d"
equation "d377 = d"
equation "d378 = d"
equation "d379 = d"
equation "d380 = d"
equation "d381 = d"
equation "d382 = d"
equation "d383 = d"
equation "d384 = d"
equation "d385 = d"
equation "d386 = d"
equation "d387 = d"
equation "d388 = d"
equation "d389 = d"
equation "d390 = d"
equation "d391 = d"
equation "d392 = d"
equation "d393 = d"
equation "d394 = d"
equation "d395 = d"
equation "d396 = d"
equation "d397 = d"
equation "d398 = d"
equation "d399 = d"
equation "d400 = d"
equation "d401 = d"
equation "d402 = d"
equation "d403 = d"
equation "d404 = d"
equation "d405 = d"
equation "d406 = d"
equation "d407 = d"
equation "d408 = d"
equation "d409 = d"
equation "d410 = d"
equation "d411 = d"
equation "d412 = d"
equation "d413 = d"
equation "d414 = d"
equation "d415 = d"
equation "d416 = d"
equation "d417 = d"
equation "d418 = d"
equation "d419 = d"
equation "d420 = d"
equation "d421 = d"
equation "d422 = d"
equation "d423 = d"
equation "d424 = d"
equation "d425 = d"
equation "d426 = d"
equation "d427 = d"
equation "d428 = d"
equation "d429 = d"
equation "d430 = d"
equation "d431 = d"
equation "d432 = d"
equation "d433 = d"
equation "d434 = d"
equation "d435 = StockHeight"
named bodies: "diamond sword body", "board"
